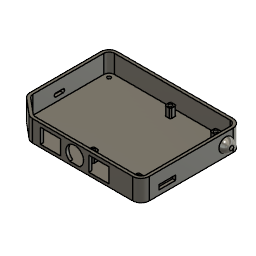
Main Casing (Autodesk Fusion 360 design; units mm, degrees)
Autodesk Fusion 360 part; units mm, degrees
derive "DerivedContext1" from "mds-0027 v11"
derive "DerivedContext2" from "mds-0027 v11"
sketch "Sketch1" plane through (0, 0, 0) normal (0, 1, 0) x (1, 0, 0)
sketch "Sketch2" plane through (0, 0, 0) normal (0, 1, 0) x (1, 0, 0)
  line L0 (47.5, 39.5) -> (45.5365, 39.5)
  line L1 (52.5365, 32.5) -> (52.5365, 33)
  line L2 (45.5365, 39.5) -> (-52.5462, 39.5)
  line L3 (-59.5462, 32.5) -> (-59.5462, -27.534)
  line L4 (-39.4265, -45.5549) -> (45.5365, -45.5549)
  line L5 (52.5365, -38.5549) -> (52.5365, 32.5)
  arc A0 (-52.5462, 39.5) -> (-59.5462, 32.5) centre (-52.5462, 32.5) ccw
  arc A1 (45.5365, -45.5549) -> (52.5365, -38.5549) centre (45.5365, -38.5549) ccw
  line L6 (-57.0487, -32.8938) -> (-43.9289, -43.9148)
  arc A2 (-43.9289, -43.9148) -> (-39.4265, -45.5549) centre (-39.4265, -38.5549) ccw
  arc A3 (-59.5462, -27.534) -> (-57.0487, -32.8938) centre (-52.5462, -27.534) ccw
  arc A4 (52.5365, 32.5) -> (45.5365, 39.5) centre (45.5365, 32.5) ccw
  line L7 (-57.0462, 32.5) -> (-57.0462, -27.534)
  arc A5 (-57.0462, -27.534) -> (-55.4406, -30.9796) centre (-52.5462, -27.534) ccw
  line L8 (-55.4406, -30.9796) -> (-42.3209, -42.0006)
  arc A6 (-42.3209, -42.0006) -> (-39.4265, -43.0549) centre (-39.4265, -38.5549) ccw
  line L9 (-39.4265, -43.0549) -> (45.5365, -43.0549)
  arc A7 (45.5365, -43.0549) -> (50.0365, -38.5549) centre (45.5365, -38.5549) ccw
  line L10 (50.0365, -38.5549) -> (50.0365, 32.5)
  arc A8 (50.0365, 32.5) -> (45.5365, 37) centre (45.5365, 32.5) ccw
  line L11 (45.5365, 37) -> (-52.5462, 37)
  arc A9 (-52.5462, 37) -> (-57.0462, 32.5) centre (-52.5462, 32.5) ccw
  dimension "d2" = 7
  dimension "d3" = 7
  dimension "d9" = 7
  dimension "d10" = 7
  dimension "d18" = -2.5
  dimension "d24" = 7
  constraint horizontal L0
  constraint perpendicular L0 L1
  constraint horizontal L2
  constraint vertical L3
  constraint horizontal L4
  constraint vertical L5
  constraint tangent L2 A0
  constraint tangent L3 A0
  constraint tangent L5 A1
  constraint tangent L4 A1
  constraint tangent L6 A2
  constraint tangent L4 A2
  constraint tangent L3 A3
  constraint tangent L6 A3
  constraint tangent L2 A4
  constraint tangent L5 A4
  measures "d2" radius of A0
  measures "d3" radius of A1
  measures "d9" radius of A2
  measures "d10" radius of A3
  measures "d24" radius of A4
extrude "Extrude1" add sketch "Sketch2" along normal blind 18 contours L2 L3 L4 L5 A0 A1 L6 A2 A3 A4 | L7 A5 L8 A6 L9 A7 L10 A8 L11 A9 makes body 1
shell "Shell1" thickness 2.5 removed faces 1 at (-15.4787, 18, -11.1484) on bodies 1
sketch "Sketch3" plane through (0, 0, 45.5549) normal (0, 0, 1) x (1, 0, 0)
  line L0 (-39.4265, 0) -> (45.5365, 0)
  line L1 (45.5365, 0) -> (45.5365, 18)
  line L2 (45.5365, 18) -> (-39.4265, 18)
  line L3 (-39.4265, 18) -> (-39.4265, 0)
  line L4 (-15.6, 15) -> (-32.6, 15)
  line L5 (-32.6, 15) -> (-32.6, 2.5)
  line L6 (-32.6, 2.5) -> (-15.6, 2.5)
  line L7 (-15.6, 2.5) -> (-15.6, 15)
  line L8 (-15.6, 15) -> (8.4, 15) construction
  line L9 (8.4, 15) -> (25.4, 15)
  line L10 (25.4, 15) -> (25.4, 2.5)
  line L11 (25.4, 2.5) -> (8.4, 2.5)
  line L12 (8.4, 2.5) -> (8.4, 15)
  line L13 (-15.6, 8.75) -> (8.4, 8.75) construction
  line L14 (-3.6, 17.5) -> (-3.6, 0)
  circle A0 centre (-3.6, 8.75) radius 7.5
  line L15 (-15.6, 2.5) -> (8.4, 2.5)
  point P0 (-24.4323, 9)
  point P1 (16.9136, 9)
  point P2 (-3.6, 8.75)
  dimension "d54" = 17
  dimension "d55" = 12.5
  dimension "d56" = 24
  dimension "d57" = 17
  dimension "d58" = 12.5
  dimension "d59" = 15
  constraint horizontal L4
  constraint vertical L5
  constraint horizontal L6
  constraint vertical L7
  constraint perpendicular L7 L8
  constraint horizontal L9
  constraint vertical L10
  constraint horizontal L11
  constraint vertical L12
  constraint midpoint L7 L13.start
  constraint midpoint L12 L13.end
  constraint midpoint L14 P2
  constraint coincident L13 P2
  constraint coincident L0 L14.end
  constraint perpendicular L0 L14
  constraint coincident P2 A0.centre
  measures "d54" distance of L4.start L4.end
  measures "d55" distance of L4.start L6.end
  measures "d56" distance of L4.start L8.end
  measures "d57" distance of L8.end L9.end
  measures "d58" distance of L8.end L11.end
  measures "d59" diameter of A0
extrude "Extrude2" cut sketch "Sketch3" against normal blind 6 contours L4 L5 L6 L7 | L9 L10 L11 L12 | L14 A0 L15 | L14 A0 L15 picked at (-3.2442, 11.6412) picked at (-3.9538, 11.6415) bodies 1
sketch "Sketch4" plane through (52.5365, 0, 0) normal (1, 0, 0) x (0, 0, -1)
  line L0 (-38.5549, 0) -> (32.5, 0)
  line L1 (32.5, 18) -> (-38.5549, 18)
  line L2 (-38.5549, 18) -> (-38.5549, 0)
  line L3 (20.5, 0) -> (20.5, 18)
  line L4 (31.9, 0) -> (31.9, 18)
  line L5 (20.5, 9) -> (31.9, 9)
  circle A0 centre (26.2, 9) radius 5.7
  circle A1 centre (26.2, 9) radius 1.75
  line L6 (32.5, 0) -> (32.5, 18)
  dimension "d11" = 3.5
  constraint coincident L0 L3.start
  constraint coincident L1 L3.end
  constraint perpendicular L1 L3
  constraint coincident L0 L4.start
  constraint coincident L1 L4.end
  constraint perpendicular L1 L4
  constraint midpoint L3 L5.start
  constraint midpoint L4 L5.end
  constraint midpoint L5 A0.centre
  constraint coincident L5.end A0
  constraint concentric A0 A1
  measures "d11" diameter of A1
extrude "Extrude3" add sketch "Sketch4" along normal blind 5 separate body contours L5 A0 A1 | L5 A0 A1 makes body 2
fillet "Fillet1" radius 5.5 1 edges at (57.5365, 6.9388, -20.8857) on bodies 2
sketch "Sketch5" plane through (0, 2.5, 0) normal (0, 1, 0) x (-1, 0, 0)
  arc A0 (57.0462, 27.534) -> (55.4406, 30.9796) centre (52.5462, 27.534) ccw
  line L0 (55.4406, 30.9796) -> (42.3209, 42.0006)
  arc A1 (42.3209, 42.0006) -> (39.4265, 43.0549) centre (39.4265, 38.5549) ccw
  line L1 (15.6, 43.0549) -> (7.7458, 43.0549)
  arc A2 (-45.5365, 43.0549) -> (-50.0365, 38.5549) centre (-45.5365, 38.5549) ccw
  line L2 (-50.0365, 38.5549) -> (-50.0365, -32.5)
  line L3 (-45.5365, -37) -> (52.5462, -37)
  arc A3 (52.5462, -37) -> (57.0462, -32.5) centre (52.5462, -32.5) ccw
  line L4 (57.0462, -32.5) -> (57.0462, 27.534)
  circle A4 centre (52.5462, -32.5) radius 1.5
  circle A5 centre (-45.5365, -32.5) radius 1.5
  circle A6 centre (-45.5365, 38.5549) radius 1.5
  arc A7 (-50.0365, -32.5) -> (-45.5365, -37) centre (-45.5365, -32.5) ccw
  line L5 (-8.4, 43.0549) -> (-8.4, 45.5549)
  line L6 (7.7458, 45.5549) -> (-0.5458, 45.5549)
  line L7 (-25.4, 45.5549) -> (-25.4, 43.0549)
  line L8 (-25.4, 43.0549) -> (-45.5365, 43.0549)
  line L9 (39.4265, 43.0549) -> (32.6, 43.0549)
  line L10 (32.6, 43.0549) -> (32.6, 45.5549)
  line L11 (32.6, 45.5549) -> (15.6, 45.5549)
  line L12 (15.6, 45.5549) -> (15.6, 43.0549)
  line L13 (7.7458, 43.0549) -> (7.7458, 45.5549)
  line L14 (-0.5458, 45.5549) -> (-0.5458, 43.0549)
  line L15 (-0.5458, 43.0549) -> (-8.4, 43.0549)
  line L16 (-8.4, 45.5549) -> (-25.4, 45.5549)
  dimension "d19" = 3
  dimension "d20" = 3
  dimension "d21" = 3
  constraint concentric A3 A4
  constraint concentric A2 A6
  measures "d19" diameter of A4
  measures "d20" diameter of A5
  measures "d21" diameter of A6
extrude "Extrude4" cut sketch "Sketch5" against normal blind 5 contours A4 | A5 | A6 bodies 1
sketch "Sketch6" plane through (0, 2.5, 0) normal (0, 1, 0) x (-1, 0, 0)
  circle A0 centre (52.5462, -32.5) radius 1.5
  circle A1 centre (-45.5365, -32.5) radius 1.5
  circle A2 centre (-45.5365, 38.5549) radius 1.5
  arc A3 (-50.0365, -32.5) -> (-45.5365, -37) centre (-45.5365, -32.5) ccw
  line L0 (-45.5365, -37) -> (52.5462, -37)
  arc A4 (52.5462, -37) -> (57.0462, -32.5) centre (52.5462, -32.5) ccw
  line L1 (57.0462, -32.5) -> (57.0462, 27.534)
  arc A5 (57.0462, 27.534) -> (55.4406, 30.9796) centre (52.5462, 27.534) ccw
  line L2 (55.4406, 30.9796) -> (42.3209, 42.0006)
  arc A6 (42.3209, 42.0006) -> (39.4265, 43.0549) centre (39.4265, 38.5549) ccw
  line L3 (15.6, 43.0549) -> (7.7458, 43.0549)
  arc A7 (-45.5365, 43.0549) -> (-50.0365, 38.5549) centre (-45.5365, 38.5549) ccw
  line L4 (-50.0365, 38.5549) -> (-50.0365, -32.5)
  line L5 (-2.9802, -32.9604) -> (-1.7802, -32.9604)
  arc A8 (-1.7802, -32.9604) -> (1.0198, -30.1604) centre (-1.7802, -30.1604) ccw
  arc A9 (1.0198, 34.7396) -> (-1.7802, 37.5396) centre (-1.7802, 34.7396) ccw
  line L6 (-42.2802, 35.0396) -> (-42.2802, 36.5396)
  line L7 (-1.4802, 35.0396) -> (1.0198, 35.0396)
  line L8 (-38.2802, 37.5396) -> (-39.4802, 37.5396)
  line L9 (-42.2802, -30.6544) -> (-42.2802, 35.2335) construction
  line L10 (1.0198, -30.4604) -> (1.0198, -30.1604)
  line L11 (-39.7802, -32.9604) -> (-39.7802, -30.4604)
  line L12 (-42.2802, 37.5396) -> (-39.7802, 37.5396)
  line L13 (1.0198, 37.5396) -> (-1.4802, 37.5396)
  line L14 (-41.2802, -32.9604) -> (-39.7802, -32.9604)
  line L15 (0.0198, -32.9604) -> (-1.4802, -32.9604)
  line L16 (-1.4802, -32.9604) -> (-1.4802, -30.4604)
  circle A10 centre (-1.4802, -30.4604) radius 1.5
  line L17 (-1.4802, 37.5396) -> (-1.4802, 35.0396)
  line L18 (-39.7802, 35.0396) -> (-42.2802, 35.0396)
  line L19 (1.0198, 35.0396) -> (1.0198, 34.7396)
  line L20 (-42.2802, -30.4604) -> (-42.2802, -31.9604)
  line L21 (-39.7802, 37.5396) -> (-39.7802, 35.0396)
  circle A11 centre (-39.7802, 35.0396) radius 1.5
  circle A12 centre (-39.7802, -30.4604) radius 1.5
  line L22 (-42.2802, -30.1604) -> (-42.2802, -28.9604)
  line L23 (-1.4802, -30.4604) -> (1.0198, -30.4604)
  arc A13 (-42.2802, -30.1604) -> (-39.4802, -32.9604) centre (-39.4802, -30.1604) ccw
  arc A14 (-39.4802, 37.5396) -> (-42.2802, 34.7396) centre (-39.4802, 34.7396) ccw
  line L24 (-39.7802, -30.4604) -> (-42.2802, -30.4604)
  line L25 (1.0198, 33.5396) -> (1.0198, 37.5396)
  circle A15 centre (-1.4802, 35.0396) radius 1.5
  line L26 (-41.2802, 37.5396) -> (-37.2802, 37.5396)
  line L27 (-37.2802, 36.5396) -> (-37.2802, 33.5396)
  line L28 (-38.2802, 32.5396) -> (-41.2802, 32.5396)
  line L29 (-42.2802, 33.5396) -> (-42.2802, 37.5396)
  line L30 (-42.2802, 37.5396) -> (-37.2802, 32.5396) construction
  line L31 (-37.2802, 37.5396) -> (-42.2802, 32.5396) construction
  line L32 (-2.9802, 37.5396) -> (0.0198, 37.5396)
  line L33 (1.0198, 36.5396) -> (1.0198, 32.5396)
  line L34 (0.0198, 32.5396) -> (-2.9802, 32.5396)
  line L35 (-3.9802, 33.5396) -> (-3.9802, 36.5396)
  line L36 (-3.9802, 37.5396) -> (1.0198, 32.5396) construction
  line L37 (1.0198, 37.5396) -> (-3.9802, 32.5396) construction
  line L38 (-2.9802, -27.9604) -> (0.0198, -27.9604)
  line L39 (1.0198, -28.9604) -> (1.0198, -32.9604)
  line L40 (1.0198, -32.9604) -> (-3.9802, -32.9604)
  line L41 (-3.9802, -31.9604) -> (-3.9802, -28.9604)
  line L42 (-3.9802, -27.9604) -> (1.0198, -32.9604) construction
  line L43 (1.0198, -27.9604) -> (-3.9802, -32.9604) construction
  line L44 (-41.2802, -27.9604) -> (-38.2802, -27.9604)
  line L45 (-37.2802, -28.9604) -> (-37.2802, -31.9604)
  line L46 (-38.2802, -32.9604) -> (-42.2802, -32.9604)
  line L47 (-42.2802, -32.9604) -> (-42.2802, -27.9604)
  line L48 (-42.2802, -27.9604) -> (-37.2802, -32.9604) construction
  line L49 (-37.2802, -27.9604) -> (-42.2802, -32.9604) construction
  arc A16 (1.0198, -28.9604) -> (0.0198, -27.9604) centre (0.0198, -28.9604) ccw
  arc A17 (-2.9802, -27.9604) -> (-3.9802, -28.9604) centre (-2.9802, -28.9604) ccw
  arc A18 (-3.9802, -31.9604) -> (-2.9802, -32.9604) centre (-2.9802, -31.9604) ccw
  arc A19 (0.0198, -32.9604) -> (1.0198, -31.9604) centre (0.0198, -31.9604) ccw
  arc A20 (-37.2802, -28.9604) -> (-38.2802, -27.9604) centre (-38.2802, -28.9604) ccw
  arc A21 (-38.2802, -32.9604) -> (-37.2802, -31.9604) centre (-38.2802, -31.9604) ccw
  arc A22 (-42.2802, -31.9604) -> (-41.2802, -32.9604) centre (-41.2802, -31.9604) ccw
  arc A23 (-41.2802, -27.9604) -> (-42.2802, -28.9604) centre (-41.2802, -28.9604) ccw
  arc A24 (1.0198, 36.5396) -> (0.0198, 37.5396) centre (0.0198, 36.5396) ccw
  arc A25 (0.0198, 32.5396) -> (1.0198, 33.5396) centre (0.0198, 33.5396) ccw
  arc A26 (-3.9802, 33.5396) -> (-2.9802, 32.5396) centre (-2.9802, 33.5396) ccw
  arc A27 (-2.9802, 37.5396) -> (-3.9802, 36.5396) centre (-2.9802, 36.5396) ccw
  arc A28 (-37.2802, 36.5396) -> (-38.2802, 37.5396) centre (-38.2802, 36.5396) ccw
  arc A29 (-38.2802, 32.5396) -> (-37.2802, 33.5396) centre (-38.2802, 33.5396) ccw
  arc A30 (-42.2802, 33.5396) -> (-41.2802, 32.5396) centre (-41.2802, 33.5396) ccw
  arc A31 (-41.2802, 37.5396) -> (-42.2802, 36.5396) centre (-41.2802, 36.5396) ccw
  line L50 (-8.4, 43.0549) -> (-8.4, 45.5549)
  line L51 (7.7458, 45.5549) -> (-0.5458, 45.5549)
  line L52 (-25.4, 45.5549) -> (-25.4, 43.0549)
  line L53 (-25.4, 43.0549) -> (-45.5365, 43.0549)
  line L54 (39.4265, 43.0549) -> (32.6, 43.0549)
  line L55 (32.6, 43.0549) -> (32.6, 45.5549)
  line L56 (32.6, 45.5549) -> (15.6, 45.5549)
  line L57 (15.6, 45.5549) -> (15.6, 43.0549)
  line L58 (7.7458, 43.0549) -> (7.7458, 45.5549)
  line L59 (-0.5458, 45.5549) -> (-0.5458, 43.0549)
  line L60 (-0.5458, 43.0549) -> (-8.4, 43.0549)
  line L61 (-8.4, 45.5549) -> (-25.4, 45.5549)
  point P0 (-42.2802, 2.2896)
  point P1 (1.0198, -32.9604)
  point P2 (-42.2802, 37.5396)
  point P3 (-39.7802, 35.0396)
  point P4 (-1.4802, 35.0396)
  point P5 (-1.4802, -30.4604)
  point P6 (-39.7802, -30.4604)
  dimension "d30" = 3
  dimension "d31" = 2.5
  dimension "d32" = 2.5
  dimension "d33" = 3
  dimension "d34" = 2.5
  dimension "d35" = 2.5
  dimension "d36" = 3
  dimension "d37" = 2.5
  dimension "d38" = 2.5
  dimension "d39" = 3
  dimension "d40" = 2.8
  dimension "d41" = 5
  dimension "d42" = 5
  dimension "d43" = 5
  dimension "d44" = 5
  dimension "d45" = 5
  dimension "d46" = 5
  dimension "d47" = 5
  dimension "d48" = 5
  dimension "d49" = 1
  constraint vertical L9
  constraint coincident P0 L9
  constraint parallel L9 L22
  constraint horizontal L5
  constraint vertical L25
  constraint horizontal L8
  constraint horizontal L14
  constraint vertical L11
  constraint horizontal L24
  constraint vertical L20
  constraint coincident P6 L11.end
  constraint horizontal L15
  constraint vertical L16
  constraint horizontal L23
  constraint vertical L10
  constraint coincident P5 L16.end
  constraint horizontal L13
  constraint vertical L17
  constraint horizontal L7
  constraint vertical L19
  constraint coincident P4 L7.start
  constraint horizontal L12
  constraint vertical L21
  constraint horizontal L18
  constraint vertical L6
  constraint coincident P3 L18.start
  constraint coincident P1 L10
  constraint coincident P1 L5
  constraint tangent A8 L10
  constraint tangent L5 A8
  constraint coincident P0 L22
  constraint tangent L22 A13
  constraint tangent L5 A13
  constraint equal A8 A13
  constraint coincident P2 L8
  constraint tangent L8 A14
  constraint equal A8 A14
  constraint coincident L13.start L19
  constraint coincident L13.start L8
  constraint tangent A9 L19
  constraint tangent A9 L8
  constraint equal A8 A9
  constraint horizontal L26
  constraint perpendicular L26 L27
  constraint parallel L26 L28
  constraint parallel L27 L29
  constraint coincident L30 P3
  constraint coincident L31 P3
  constraint horizontal L32
  constraint perpendicular L32 L33
  constraint parallel L32 L34
  constraint parallel L33 L35
  constraint coincident L36 P4
  constraint coincident L37 P4
  constraint horizontal L38
  constraint perpendicular L38 L39
  constraint parallel L38 L40
  constraint parallel L39 L41
  constraint coincident L42 P5
  constraint coincident L43 P5
  constraint horizontal L44
  constraint perpendicular L44 L45
  constraint parallel L44 L46
  constraint parallel L45 L47
  constraint coincident L48 P6
  constraint coincident L49 P6
  constraint coincident L43.start L39
  constraint coincident L43.start L38
  constraint tangent L39 A16
  constraint tangent L38 A16
  constraint coincident L42.start L38
  constraint coincident L42.start L41
  constraint tangent L38 A17
  constraint tangent L41 A17
  constraint equal A16 A17
  constraint coincident L40.end L41
  constraint coincident A13.end L5
  constraint tangent L41 A18
  constraint tangent L5 A18
  constraint equal A16 A18
  constraint coincident P1 L15
  constraint coincident P1 L25
  constraint tangent L15 A19
  constraint tangent L25 A19
  constraint equal A16 A19
  constraint coincident L49.start L44
  constraint coincident L49.start L45
  constraint tangent L44 A20
  constraint tangent L45 A20
  constraint equal A16 A20
  constraint coincident L48.end L45
  constraint coincident L48.end L46
  constraint tangent L45 A21
  constraint tangent L46 A21
  constraint equal A16 A21
  constraint tangent L14 A22
  constraint tangent L20 A22
  constraint equal A16 A22
  constraint coincident P2 L22
  constraint coincident L47.end L44
  constraint tangent L22 A23
  constraint tangent L44 A23
  constraint equal A16 A23
  constraint coincident L13.start L33
  constraint coincident L13.start L32
  constraint tangent L33 A24
  constraint tangent L32 A24
  constraint equal A16 A24
  constraint coincident L25 A19.end
  constraint coincident L33.end L34
  constraint tangent L25 A25
  constraint tangent L34 A25
  constraint equal A16 A25
  constraint coincident L37.end L34
  constraint coincident L37.end L35
  constraint tangent L34 A26
  constraint tangent L35 A26
  constraint equal A16 A26
  constraint coincident L36.start L32
  constraint coincident L36.start L35
  constraint tangent L32 A27
  constraint tangent L35 A27
  constraint equal A16 A27
  constraint coincident A9.end L8
  constraint coincident L26.end L27
  constraint tangent L8 A28
  constraint tangent L27 A28
  constraint equal A16 A28
  constraint coincident L30.end L27
  constraint coincident L30.end L28
  constraint tangent L27 A29
  constraint tangent L28 A29
  constraint equal A16 A29
  constraint coincident L31.end L28
  constraint coincident L31.end L29
  constraint tangent L28 A30
  constraint tangent L29 A30
  constraint equal A16 A30
  constraint coincident P2 L26
  constraint coincident P2 L6
  constraint tangent L26 A31
  constraint tangent L6 A31
  constraint equal A16 A31
  measures "d30" diameter of A12
  measures "d31" distance of P1 L15.end
  measures "d32" distance of P1 L10.start
  measures "d33" diameter of A10
  measures "d34" distance of L13.end L13.start
  measures "d35" distance of L7.end L13.start
  measures "d36" diameter of A15
  measures "d37" distance of P2 L12.end
  measures "d38" distance of P2 L6.start
  measures "d39" diameter of A11
  measures "d40" radius of A8
  measures "d41" distance of L30.end L31.end
  measures "d42" distance of L26.end L30.end
  measures "d43" distance of L33.end L37.end
  measures "d44" distance of L13.start L33.end
  measures "d45" distance of P1 L40.end
  measures "d46" distance of L43.start P1
  measures "d47" distance of L48.end L46.end
  measures "d48" distance of L49.start L48.end
  measures "d49" radius of A16
extrude "Extrude5" add sketch "Sketch6" along normal blind 7.6 contours L5 A8 L16 A10 L23 L38 L39 L40 L41 A16 A17 A18 | A8 L16 A10 L23 | A8 L15 L16 L23 L39 L40 A19 | A9 L7 L17 L25 A15 L32 L33 L34 L35 A25 A26 A27 | A9 L7 L17 A15 | A9 L7 L13 L17 L25 L32 L33 A24 | L6 L12 L18 L21 A14 L26 L29 A31 | L18 L21 A11 A14 | L8 L18 L21 A11 A14 L26 L27 L28 L29 A28 A29 A30 | L11 L14 L20 A13 L24 L46 L47 A22 | L11 A12 A13 L24 | L11 A12 L22 A13 L24 L44 L45 L46 L47 A20 A21 A23 bodies 1
sketch "Sketch7" plane through (0, 2.5, 0) normal (0, 1, 0) x (-1, 0, 0)
  line L0 (-1.4802, -32.9604) -> (-1.4802, -32.9443)
  arc A0 (-1.7802, -32.9604) -> (-1.4802, -32.9443) centre (-1.7802, -30.1604) ccw
  line L1 (-1.7802, -32.9604) -> (-2.9802, -32.9604)
  arc A1 (-3.9802, -31.9604) -> (-2.9802, -32.9604) centre (-2.9802, -31.9604) ccw
  line L2 (-3.9802, -31.9604) -> (-3.9802, -28.9604)
  arc A2 (-2.9802, -27.9604) -> (-3.9802, -28.9604) centre (-2.9802, -28.9604) ccw
  line L3 (-2.9802, -27.9604) -> (0.0198, -27.9604)
  arc A3 (1.0198, -28.9604) -> (0.0198, -27.9604) centre (0.0198, -28.9604) ccw
  line L4 (1.0198, -28.9604) -> (1.0198, -30.1604)
  arc A4 (1.0037, -30.4604) -> (1.0198, -30.1604) centre (-1.7802, -30.1604) ccw
  line L5 (1.0037, -30.4604) -> (1.0198, -30.4604)
  line L6 (1.0198, -30.4604) -> (1.0198, -31.9604)
  arc A5 (0.0198, -32.9604) -> (1.0198, -31.9604) centre (0.0198, -31.9604) ccw
  line L7 (0.0198, -32.9604) -> (-1.4802, -32.9604)
  line L8 (-37.2802, -28.9604) -> (-37.2802, -31.9604)
  arc A6 (-38.2802, -32.9604) -> (-37.2802, -31.9604) centre (-38.2802, -31.9604) ccw
  line L9 (-38.2802, -32.9604) -> (-39.4802, -32.9604)
  arc A7 (-39.7802, -32.9443) -> (-39.4802, -32.9604) centre (-39.4802, -30.1604) ccw
  line L10 (-39.7802, -32.9443) -> (-39.7802, -32.9604)
  line L11 (-39.7802, -32.9604) -> (-41.2802, -32.9604)
  arc A8 (-42.2802, -31.9604) -> (-41.2802, -32.9604) centre (-41.2802, -31.9604) ccw
  line L12 (-42.2802, -31.9604) -> (-42.2802, -30.4604)
  line L13 (-42.2802, -30.4604) -> (-42.2641, -30.4604)
  arc A9 (-42.2802, -30.1604) -> (-42.2641, -30.4604) centre (-39.4802, -30.1604) ccw
  line L14 (-42.2802, -30.1604) -> (-42.2802, -28.9604)
  arc A10 (-41.2802, -27.9604) -> (-42.2802, -28.9604) centre (-41.2802, -28.9604) ccw
  line L15 (-41.2802, -27.9604) -> (-38.2802, -27.9604)
  arc A11 (-37.2802, -28.9604) -> (-38.2802, -27.9604) centre (-38.2802, -28.9604) ccw
  circle A12 centre (52.5462, -32.5) radius 1.5
  circle A13 centre (-45.5365, -32.5) radius 1.5
  circle A14 centre (-45.5365, 38.5549) radius 1.5
  arc A15 (-50.0365, -32.5) -> (-45.5365, -37) centre (-45.5365, -32.5) ccw
  line L16 (-45.5365, -37) -> (52.5462, -37)
  arc A16 (52.5462, -37) -> (57.0462, -32.5) centre (52.5462, -32.5) ccw
  line L17 (57.0462, -32.5) -> (57.0462, 27.534)
  arc A17 (57.0462, 27.534) -> (55.4406, 30.9796) centre (52.5462, 27.534) ccw
  line L18 (55.4406, 30.9796) -> (42.3209, 42.0006)
  arc A18 (42.3209, 42.0006) -> (39.4265, 43.0549) centre (39.4265, 38.5549) ccw
  line L19 (15.6, 43.0549) -> (7.7458, 43.0549)
  arc A19 (-45.5365, 43.0549) -> (-50.0365, 38.5549) centre (-45.5365, 38.5549) ccw
  line L20 (-50.0365, 38.5549) -> (-50.0365, -32.5)
  line L21 (-39.7802, 37.5396) -> (-39.7802, 37.5234)
  arc A20 (-39.4802, 37.5396) -> (-39.7802, 37.5234) centre (-39.4802, 34.7396) ccw
  line L22 (-39.4802, 37.5396) -> (-38.2802, 37.5396)
  arc A21 (-37.2802, 36.5396) -> (-38.2802, 37.5396) centre (-38.2802, 36.5396) ccw
  line L23 (-37.2802, 36.5396) -> (-37.2802, 33.5396)
  arc A22 (-38.2802, 32.5396) -> (-37.2802, 33.5396) centre (-38.2802, 33.5396) ccw
  line L24 (-38.2802, 32.5396) -> (-41.2802, 32.5396)
  arc A23 (-42.2802, 33.5396) -> (-41.2802, 32.5396) centre (-41.2802, 33.5396) ccw
  line L25 (-42.2802, 33.5396) -> (-42.2802, 34.7396)
  arc A24 (-42.2641, 35.0396) -> (-42.2802, 34.7396) centre (-39.4802, 34.7396) ccw
  line L26 (-42.2641, 35.0396) -> (-42.2802, 35.0396)
  line L27 (-42.2802, 35.0396) -> (-42.2802, 36.5396)
  arc A25 (-41.2802, 37.5396) -> (-42.2802, 36.5396) centre (-41.2802, 36.5396) ccw
  line L28 (-41.2802, 37.5396) -> (-39.7802, 37.5396)
  line L29 (-1.4802, 37.5396) -> (0.0198, 37.5396)
  arc A26 (1.0198, 36.5396) -> (0.0198, 37.5396) centre (0.0198, 36.5396) ccw
  line L30 (1.0198, 36.5396) -> (1.0198, 35.0396)
  line L31 (1.0198, 35.0396) -> (1.0037, 35.0396)
  arc A27 (1.0198, 34.7396) -> (1.0037, 35.0396) centre (-1.7802, 34.7396) ccw
  line L32 (1.0198, 34.7396) -> (1.0198, 33.5396)
  arc A28 (0.0198, 32.5396) -> (1.0198, 33.5396) centre (0.0198, 33.5396) ccw
  line L33 (0.0198, 32.5396) -> (-2.9802, 32.5396)
  arc A29 (-3.9802, 33.5396) -> (-2.9802, 32.5396) centre (-2.9802, 33.5396) ccw
  line L34 (-3.9802, 33.5396) -> (-3.9802, 36.5396)
  arc A30 (-2.9802, 37.5396) -> (-3.9802, 36.5396) centre (-2.9802, 36.5396) ccw
  line L35 (-2.9802, 37.5396) -> (-1.7802, 37.5396)
  arc A31 (-1.4802, 37.5234) -> (-1.7802, 37.5396) centre (-1.7802, 34.7396) ccw
  line L36 (-1.4802, 37.5234) -> (-1.4802, 37.5396)
  line L37 (-8.4, 43.0549) -> (-8.4, 45.5549)
  line L38 (7.7458, 45.5549) -> (-0.5458, 45.5549)
  line L39 (-25.4, 45.5549) -> (-25.4, 43.0549)
  line L40 (-25.4, 43.0549) -> (-45.5365, 43.0549)
  line L41 (39.4265, 43.0549) -> (32.6, 43.0549)
  line L42 (32.6, 43.0549) -> (32.6, 45.5549)
  line L43 (32.6, 45.5549) -> (15.6, 45.5549)
  line L44 (15.6, 45.5549) -> (15.6, 43.0549)
  line L45 (7.7458, 43.0549) -> (7.7458, 45.5549)
  line L46 (-0.5458, 45.5549) -> (-0.5458, 43.0549)
  line L47 (-0.5458, 43.0549) -> (-8.4, 43.0549)
  line L48 (-8.4, 45.5549) -> (-25.4, 45.5549)
  line L49 (-25.4, 43.0549) -> (-8.4, 43.0549)
  line L50 (-0.5458, 43.0549) -> (7.7458, 43.0549)
  line L51 (15.6, 43.0549) -> (32.6, 43.0549)
  line L52 (-1.4802, -30.4604) -> (-11.7402, -30.4604)
  line L53 (-39.7802, -30.4604) -> (-29.5202, -30.4604)
  point P0 (-39.7802, -30.4604)
  point P1 (-1.4802, -30.4604)
  dimension "d62" = 10.26
  dimension "d63" = 10.26
  constraint coincident L39.end L40.start
  constraint coincident L37.start L47.end
  constraint coincident L46.end L47.start
  constraint coincident L19.end L45.start
  constraint coincident L19.start L44.end
  constraint coincident L41.end L42.start
  constraint coincident P1 L52.start
  constraint parallel L3 L52
  constraint coincident P0 L53.start
  constraint horizontal L53
  measures "d62" distance of P1 L52.end
  measures "d63" distance of P0 L53.end
sketch "sketch 10827" plane through (-59.5462, 0, 0) normal (-1, 0, 0) x (0, 0, 1)
  line L0 (-32.5, 0) -> (27.534, 0)
  line L1 (27.534, 0) -> (27.534, 18)
  line L2 (27.534, 18) -> (-32.5, 18)
  line L3 (-32.5, 18) -> (-32.5, 0)
  line L4 (0.5547, 8.045) -> (0.5547, 7.335)
  arc A0 (0.5547, 7.335) -> (1.8047, 6.085) centre (1.8047, 7.335) ccw
  line L5 (1.8047, 6.085) -> (8.2447, 6.085)
  arc A1 (8.2447, 6.085) -> (9.4947, 7.335) centre (8.2447, 7.335) ccw
  line L6 (9.4947, 7.335) -> (9.4947, 8.045)
  arc A2 (9.4947, 8.045) -> (8.2447, 9.295) centre (8.2447, 8.045) ccw
  line L7 (8.2447, 9.295) -> (1.8047, 9.295)
  arc A3 (1.8047, 9.295) -> (0.5547, 8.045) centre (1.8047, 8.045) ccw
  arc A4 (9.3447, 8.045) -> (8.2447, 9.145) centre (8.2447, 8.045) ccw
  line L8 (9.3447, 8.045) -> (9.3447, 7.335)
  arc A5 (8.2447, 6.235) -> (9.3447, 7.335) centre (8.2447, 7.335) ccw
  line L9 (8.2447, 6.235) -> (1.8047, 6.235)
  arc A6 (0.7047, 7.335) -> (1.8047, 6.235) centre (1.8047, 7.335) ccw
  line L10 (0.7047, 7.335) -> (0.7047, 8.045)
  arc A7 (1.8047, 9.145) -> (0.7047, 8.045) centre (1.8047, 8.045) ccw
  line L11 (1.8047, 9.145) -> (8.2447, 9.145)
  line L12 (0.3047, 8.045) -> (0.3047, 7.335)
  arc A8 (0.3047, 7.335) -> (1.8047, 5.835) centre (1.8047, 7.335) ccw
  line L13 (1.8047, 5.835) -> (8.2447, 5.835)
  arc A9 (8.2447, 5.835) -> (9.7447, 7.335) centre (8.2447, 7.335) ccw
  line L14 (9.7447, 7.335) -> (9.7447, 8.045)
  arc A10 (9.7447, 8.045) -> (8.2447, 9.545) centre (8.2447, 8.045) ccw
  line L15 (8.2447, 9.545) -> (1.8047, 9.545)
  arc A11 (1.8047, 9.545) -> (0.3047, 8.045) centre (1.8047, 8.045) ccw
  line L16 (8.2447, 6.235) -> (1.8047, 6.235)
  arc A12 (0.7047, 7.335) -> (1.8047, 6.235) centre (1.8047, 7.335) ccw
  line L17 (0.7047, 7.335) -> (0.7047, 8.045)
  arc A13 (1.8047, 9.145) -> (0.7047, 8.045) centre (1.8047, 8.045) ccw
  line L18 (1.8047, 9.145) -> (8.2447, 9.145)
  arc A14 (9.3447, 8.045) -> (8.2447, 9.145) centre (8.2447, 8.045) ccw
  line L19 (9.3447, 8.045) -> (9.3447, 7.335)
  arc A15 (8.2447, 6.235) -> (9.3447, 7.335) centre (8.2447, 7.335) ccw
extrude "Extrude6" cut sketch "sketch 10827" against normal blind 5 contours A4 L8 A5 L9 A6 L10 A7 L11 L16 A12 L17 A13 L18 A14 L19 A15 bodies 1
sketch "Sketch13" plane through (52.5365, 0, 0) normal (1, 0, 0) x (0, 0, -1)
  line L0 (-38.5549, 0) -> (32.5, 0)
  line L1 (32.5, 0) -> (32.5, 18)
  line L2 (32.5, 18) -> (-38.5549, 18)
  line L3 (-38.5549, 18) -> (-38.5549, 0)
  line L4 (-30.3, 6.9) -> (-16.3, 6.9)
  line L5 (-30.3, 5) -> (-30.3, 6.9)
  line L6 (-16.3, 5) -> (-30.3, 5)
  line L7 (-16.3, 6.9) -> (-16.3, 5)
  line L8 (-30.3, 6.9) -> (-30.3, 7.9)
  line L9 (-30.3, 5) -> (-30.3, 4)
  line L10 (-16.3, 5) -> (-16.3, 4)
  line L11 (-16.3, 4) -> (-30.3, 4)
  line L12 (-30.3, 4) -> (-30.3, 7.9)
  line L13 (-30.3, 7.9) -> (-16.3, 7.9)
  line L14 (-16.3, 7.9) -> (-16.3, 4)
  dimension "d68" = 1
  dimension "d69" = 1
  dimension "d70" = 1
  constraint coincident L4.start L5.end
  constraint perpendicular L4 L8
  constraint coincident L5.start L6.end
  constraint perpendicular L6 L9
  constraint coincident L6.start L7.end
  constraint perpendicular L6 L10
  constraint horizontal L11
  constraint vertical L12
  constraint horizontal L13
  constraint vertical L14
  measures "d68" distance of L4.start L8.end
  measures "d69" distance of L5.start L9.end
  measures "d70" distance of L6.start L10.end
sketch "sketch 11622" plane through (52.5365, 0, 0) normal (1, 0, 0) x (0, 0, -1)
  line L0 (-38.5549, 0) -> (32.5, 0)
  line L1 (32.5, 0) -> (32.5, 18)
  line L2 (32.5, 18) -> (-38.5549, 18)
  line L3 (-38.5549, 18) -> (-38.5549, 0)
  line L4 (-30.3, 6.9) -> (-16.3, 6.9)
  line L5 (-16.3, 6.9) -> (-16.3, 5)
  line L6 (-16.3, 5) -> (-30.3, 5)
  line L7 (-30.3, 5) -> (-30.3, 6.9)
  line L8 (-16.3, 6.9) -> (-16.3, 5)
  line L9 (-16.3, 5) -> (-30.3, 5)
  line L10 (-30.3, 5) -> (-30.3, 6.9)
  line L11 (-30.3, 6.9) -> (-16.3, 6.9)
extrude "Extrude7" cut sketch "Sketch13" sketch "sketch 11622" against normal blind 5 contours L4 L8 L12 L13 L14 | L6 L9 L10 L11 L12 L14 of sketch 2 contours L4 L5 L6 L7 L8 L9 L10 L11 bodies 1
